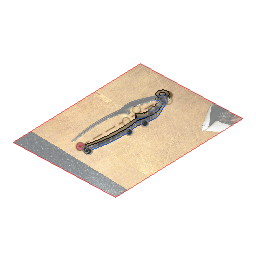
Day27 - nutcracker (Autodesk Fusion 360 design; units mm, degrees)
Autodesk Fusion 360 part; units mm, degrees
sketch "Sketch1" plane through (0, 0, 0) normal (0, 0, 1) x (1, 0, 0)
  line L0 (0, 0) -> (0, 100) construction
  spline S0 degree 5 poles (9.0149, 0.2946) (9.5097, 2.1293) (10.4161, 5.7155) (11.526, 10.8441) (12.5431, 17.2157) (13.2131, 24.5364) (13.4993, 31.3641) (13.503, 37.6645) (13.3472, 43.3984) (12.5906, 47.7828) (11.9387, 51.48) (12.4129, 55.8693) (14.3306, 61.8643) (15.2698, 67.9598) (14.3731, 73.7666) (11.8128, 79.6447) (8.9953, 84.9689) (6.8044, 89.6341) (5.3645, 93.0908) (4.6498, 94.9059) knots 0 0 0 0 0 0 0.066667 0.133333 0.2 0.266667 0.333333 0.4 0.466667 0.533333 0.6 0.666667 0.733333 0.8 0.866667 0.933333 1 1 1 1 1 1
  line L1 (13.8572, 33.744) -> (12.7172, 50.3398)
  line L2 (11.2146, 50.209) -> (15.81, 68.631)
  line L3 (9.8225, 81.77) -> (-0.5229, 108.0417)
  line L4 (5.6835, -12.0589) -> (12.3463, 12.648)
  spline S1 degree 3 poles (6.1527, 0.8579) (8.0675, 7.6092) (9.0398, 13.603) (9.4896, 19.1536) (9.831, 23.3656) (9.9018, 27.3513) (9.9036, 31.1272) (9.9051, 34.2745) (9.8709, 37.3072) (9.7974, 40.0094) (9.74, 42.1228) (9.6302, 43.9688) (9.4489, 45.5961) (9.2467, 47.4119) (8.9428, 49.0121) (8.7968, 50.8779) (8.6679, 52.5239) (8.7284, 54.3696) (9.0797, 56.3408) (9.5833, 59.1668) (10.616, 62.2509) (11.1296, 65.104) (11.5365, 67.3641) (11.6278, 69.4511) (11.3214, 71.5341) (10.9664, 73.9477) (10.0615, 76.434) (8.7213, 79.3685) (7.2561, 82.5765) (5.3218, 86.3153) (3.4307, 90.7989) (2.8908, 92.0789) (2.3528, 93.4174) (1.821, 94.8124) knots 0 0 0 0 0.148863 0.148863 0.148863 0.261826 0.261826 0.261826 0.355983 0.355983 0.355983 0.429622 0.429622 0.429622 0.511788 0.511788 0.511788 0.58428 0.58428 0.58428 0.68821 0.68821 0.68821 0.770538 0.770538 0.770538 0.865935 0.865935 0.865935 0.970227 0.970227 0.970227 1 1 1 1
  arc A0 (6.1527, 0.8579) -> (9.0149, 0.2946) centre (7.6033, 0.6752) ccw
  arc A1 (8.7847, 53.9472) -> (3.995, 58.2753) centre (1.3978, 50.5867) ccw
  arc A2 (3.995, 58.2753) -> (7.5301, 72.382) centre (-4.0381, 67.7847) ccw
  spline S2 degree 5 poles (7.5301, 72.382) (7.2078, 73.1932) (6.6862, 74.6934) (6.2732, 76.5779) (6.2974, 78.5387) (6.5279, 80.9356) (6.1673, 83.6473) (5.2089, 86.5963) (4.1969, 89.0538) (3.5975, 90.4055) knots 0 0 0 0 0 0 0.2 0.4 0.6 0.8 1 1 1 1 1 1
  line L5 (4.9973, 87.2484) -> (2.1976, 93.5626)
  circle A3 centre (0, 93.0778) radius 2.5394
  circle A4 centre (0, 93.0778) radius 5.4756
  arc A5 (4.8755, 87.3516) -> (2.4831, 88.1976) centre (3.2771, 86.6371) ccw
  dimension "d1" = 100
extrude "Extrude1" add sketch "Sketch1" along normal blind 5 and the other way blind 0 contours S0 S1 A0 L5 A4 | S1 A1 A2 S2 | S1 S2 L5 A4 | S0 L3 A4 | S0 L3 A4 | S1 S2 A4 A5 | S2 L5 A4 | S1 L5 A3 | L3 S1 L5 A4
sketch "Sketch2" plane through (0, 0, 0) normal (0, 0, 1) x (1, 0, 0)
  line L0 (7.0779, 63.9956) -> (8.642, 64.3966)
  line L1 (8.642, 64.3966) -> (7.4926, 65.328)
  line L2 (7.4926, 65.328) -> (7.0779, 63.9956)
  circle A0 centre (4.7194, 76.6741) radius 2.9083
extrude "Extrude2" cut sketch "Sketch2" along normal through all and the other way through all contours L0 L1 L2
pattern_path "PathPattern1" count 6 spacing 1.6994 from (8.0631, 64.8657, 5) along 2 edges at (6.3666, 79.1921, 5) (8.379, 68.6651, 5) of "Extrude2"
extrude "Extrude3" cut sketch "Sketch2" along normal through all and the other way through all contours A0
